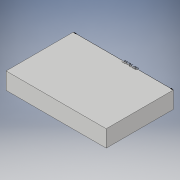
# Autodesk Inventor part: Part1
Saved by Autodesk Inventor 2018 (Build 220112000, 112)
## iProperties
Created: 2018-12-04
Part Number: Part1
Material: Generic
Document SubType Name: Modeling
Designer: 10043883
Density: 1 g/cm^3
Appearance: Default
Author: 10043883
Autodesk Inventor part; units mm, degrees
ref_plane "YZ Plane" through (0, 0, 0) normal (1, 0, 0) x (0, 1, 0)
ref_plane "XZ Plane" through (0, 0, 0) normal (0, 1, 0) x (-1, 0, 0)
ref_plane "XY Plane" through (0, 0, 0) normal (0, 0, 1) x (1, 0, 0)
sketch "Sketch2" plane through (0, 0, 0) normal (0, 1, 0) x (-1, 0, 0)
  line L0 (4.6641, 30486.7325) -> (-90825.7359, 30486.7325)
  line L1 (-90825.7359, 30486.7325) -> (-90825.7359, -30473.2675)
  line L2 (-90825.7359, -30473.2675) -> (4.6641, -30473.2675)
  line L3 (4.6641, -30473.2675) -> (4.6641, 30486.7325)
  point P0 (0, 0)
  dimension "d2" = 90830.4
  dimension "d3" = 60960
  constraints: 8 end point, 2 parallel, 1 horizontal, 1 perpendicular
  measures "d2" distance of L2.end L1.end
  measures "d3" distance of L1.end L0.end
extrude "Extrusion1" add sketch "Sketch2" along normal blind 15240
body "Solid1"
